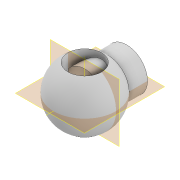
# Autodesk Inventor part: LowerarmP
Saved by Autodesk Inventor 2021 (Build 250183000, 183)
## iProperties
Created: 2020-12-19
Part Number: LowerarmP
Material: 一般
Document SubType Name: Modeling
Designer: Tazaki
Density: 2.55349 g/cm^3
Appearance: 既定
Mass: 500 g
Surface Area: 266.995 cm^2
Volume: 195.81 cm^3
Author: Tazaki
Autodesk Inventor part; units mm, degrees
ref_plane "YZ Plane" through (0, 0, 0) normal (1, 0, 0) x (0, 1, 0)
sketch "スケッチ1" plane through (0, 0, 0) normal (0, 0, 1) x (1, 0, 0)
  arc A0 (0, 37.5) -> (0, -37.5) centre (0, 0) ccw
  line L0 (0, 37.5) -> (0, -37.5)
  dimension "d0" = 75
  constraints: 2 end point, 2 point on circle, 1 centre point, 1 coincident, 1 vertical
  measures "d0" diameter of A0
revolve "回転1" add sketch "スケッチ1" angle 360 about axis through (0, 37.5, 0) along (0, -1, 0)
sketch "スケッチ2" plane through (0, 0, 0) normal (0, 1, 0) x (-1, 0, 0)
  circle A0 centre (0, 0) radius 20
  dimension "d2" = 40
  constraints: 1 centre point, 1 coincident
  measures "d2" diameter of A0
extrude "押し出し1" cut sketch "スケッチ2" along normal mid plane 100
sketch "スケッチ3" plane through (0, 0, 0) normal (0, 0, 1) x (1, 0, 0)
  circle A0 centre (0, 0) radius 25
  dimension "d5" = 50
  constraints: 1 centre point, 1 coincident
  measures "d5" diameter of A0
extrude "押し出し2" add sketch "スケッチ3" against normal blind 50
